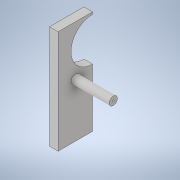
# Autodesk Inventor part: hook
Saved by Autodesk Inventor 2021 (Build 250183000, 183)
## iProperties
Created: 2020-10-22
Part Number: hook
Material: Generic
Document SubType Name: Modeling
Designer: User
Density: 1 g/cm^3
Appearance: Default
Author: User
Autodesk Inventor part; units mm, degrees
ref_plane "YZ Plane" through (0, 0, 0) normal (1, 0, 0) x (0, 1, 0)
ref_plane "XZ Plane" through (0, 0, 0) normal (0, 1, 0) x (-1, 0, 0)
ref_plane "XY Plane" through (0, 0, 0) normal (0, 0, 1) x (1, 0, 0)
sketch "Sketch1" plane through (0, 0, 0) normal (1, 0, 0) x (0, 1, 0)
  line L0 (0, 0) -> (76.2, 0)
  line L1 (76.2, 0) -> (76.2, -25.4)
  line L2 (76.2, -25.4) -> (0, -25.4)
  line L3 (0, -25.4) -> (0, 0)
  arc A0 (74.6125, -25.4) -> (42.8625, -25.4) centre (58.7375, -25.4) ccw
  dimension "d0" = 76.2
  dimension "d1" = 25.4
  dimension "d2" = 31.75
  dimension "d3" = 15.875
  dimension "d20" = 1.5875
  constraints: 8 end point, 2 parallel, 2 point on circle, 2 point on line, 1 centre point, 1 horizontal, 1 perpendicular
  measures "d0" distance of L1.end L2.end
  measures "d1" distance of L0.end L1.end
  measures "d2" distance of A0.start A0.end
  measures "d3" radius of A0
  measures "d20" distance from line of L1 A0.start
extrude "Extrusion1" add sketch "Sketch1" along normal blind 6.35 contours L0 L1 L2 A0 L3
sketch "Sketch2" plane through (0, 0, -25.4) normal (0, -1, 0) x (1, 0, 0)
  line L0 (3.175, 21.59) -> (3.175, 3.81) construction
  line L1 (1.905, 20.32) -> (1.905, 5.08)
  line L2 (4.445, 5.08) -> (4.445, 20.32)
  arc A0 (4.445, 20.32) -> (1.905, 20.32) centre (3.175, 20.32) ccw
  arc A1 (1.905, 5.08) -> (4.445, 5.08) centre (3.175, 5.08) ccw
  line L3 (6.35, 25.4) -> (6.35, 0) projected
  line L4 (0, 25.4) -> (6.35, 25.4) projected
  point P0 (3.175, 12.7)
  dimension "d6" = 2.54
  dimension "d7" = 25.4
  dimension "d8" = 12.7
  dimension "d9" = 8.89
  constraints: 8 end point, 6 point on circle, 4 tangent, 2 centre point, 2 point on line, 1 midpoint, 1 parallel, 1 vertical
  measures "d6" diameter of A1
  measures "d7" distance of L3.start L3.end
  measures "d8" distance from line of L4 point (3.175, 12.7)
  measures "d9" distance of point (3.175, 12.7) L0.start
extrude "Extrusion2" cut sketch "Sketch2" against normal blind 38.1
sketch "Sketch4" plane through (6.35, 0, 0) normal (1, 0, 0) x (0, 0, -1)
  line L0 (5.08, 0) -> (5.08, 38.1) projected
  line L1 (0, 0) -> (25.4, 0) projected
  line L2 (25.4, 0) -> (25.4, 42.8625) projected
  arc A0 (25.4, 74.6125) -> (25.4, 42.8625) centre (25.4, 58.7375) ccw projected
  line L3 (25.4, 76.2) -> (0, 76.2) projected
  line L4 (0, 76.2) -> (0, 0) projected
  circle A1 centre (12.7, 39.7791) radius 0.635
  circle A2 centre (12.7, 39.7791) radius 3.048
  line L5 (25.4, 74.6125) -> (25.4, 76.2) projected
  dimension "d16" = 1.27
  dimension "d17" = 6.096
  constraints: 2 centre point, 1 coincident
  measures "d16" diameter of A1
  measures "d17" diameter of A2
extrude "Extrusion4" add sketch "Sketch4" along normal blind 27.94 contours A2
equation "\"d8\" = 0.5 * d7"
body "Solid1"
